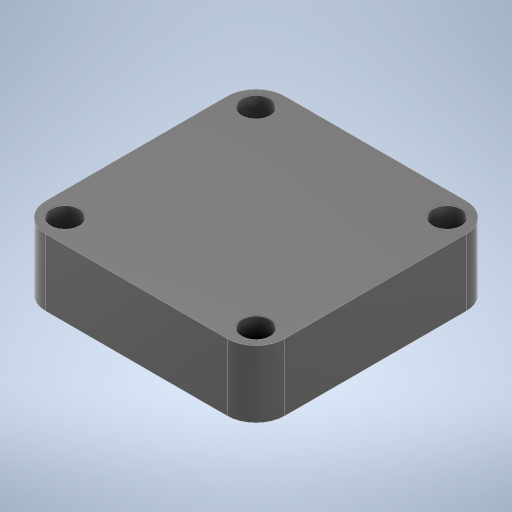
# Autodesk Inventor part: YDM2507C12F
Saved by Autodesk Inventor 2024.2 (Build 282272000, 272)
## iProperties
Created: 2024-01-24
Part Number: YDM2507C12F
Material: Acetal Resin, Black
Document SubType Name: Modeling
Designer: Masato Kubotera
Density: 1.425 g/cm^3
Appearance: Smooth - Black
Vendor: YCCFAN Technology
Author: Masato Kubotera
Autodesk Inventor part; units mm, degrees
ref_plane "YZ Plane" through (0, 0, 0) normal (1, 0, 0) x (0, 1, 0)
ref_plane "XZ Plane" through (0, 0, 0) normal (0, 1, 0) x (-1, 0, 0)
ref_plane "XY Plane" through (0, 0, 0) normal (0, 0, 1) x (1, 0, 0)
sketch "Sketch1" plane through (0, 0, 0) normal (0, 0, 1) x (1, 0, 0)
  line L0 (12.5, -12.5) -> (-12.5, -12.5)
  line L1 (-12.5, -12.5) -> (-12.5, 12.5)
  line L2 (-12.5, 12.5) -> (12.5, 12.5)
  line L3 (12.5, 12.5) -> (12.5, -12.5)
  line L4 (12.5, -12.5) -> (-12.5, 12.5) construction
  line L5 (-12.5, -12.5) -> (12.5, 12.5) construction
  line L6 (10, -10) -> (-10, -10) construction
  line L7 (-10, -10) -> (-10, 10) construction
  line L8 (-10, 10) -> (10, 10) construction
  line L9 (10, 10) -> (10, -10) construction
  line L10 (10, -10) -> (-10, 10) construction
  line L11 (-10, -10) -> (10, 10) construction
  point P0 (0, 0)
  dimension "d0" = 25
  dimension "d1" = 25
  dimension "d2" = 20
  dimension "d3" = 20
  constraints: 24 end point, 4 midpoint, 4 parallel, 2 horizontal, 2 perpendicular
  measures "d0" distance of L1.end L2.end
  measures "d1" distance of L0.end L1.end
  measures "d2" distance of L7.end L8.end
  measures "d3" distance of L6.end L7.end
extrude "Extrusion1" add sketch "Sketch1" along normal blind 7
fillet "Fillet1" radius 3 4 edges at (12.5, -12.5, 3.5) (-12.5, -12.5, 3.5) (12.5, 12.5, 3.5) (-12.5, 12.5, 3.5)
hole "Hole1" at (10, -10, 0) at (10, 10, 0) at (-10, 10, 0) at (-10, -10, 0) direction (0, 0, 1) diameter 3 end through all
body "Solid1"
